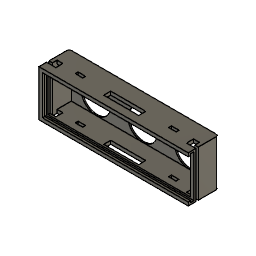
Canal - base v22 (Autodesk Fusion 360 design; units mm, degrees)
Autodesk Fusion 360 part; units mm, degrees
sketch "Esquisse1" plane through (0, 0, 0) normal (0, 1, 0) x (1, 0, 0)
  line L0 (-18.0113, -0.0987) -> (45.9887, -0.0987)
  line L1 (45.9887, -0.0987) -> (45.9887, -19.8487)
  line L2 (45.9887, -19.8487) -> (-18.0113, -19.8487)
  line L3 (-18.0113, -19.8487) -> (-18.0113, -0.0987)
  dimension "d1" = 64
  dimension "d2" = 19.75
  constraint horizontal L0
  constraint vertical L1
  constraint horizontal L2
  constraint vertical L3
  measures "d1" distance of L1 L3
  measures "d2" distance of L0 L2
extrude "Extrusion1" add sketch "Esquisse1" along normal blind 13
shell "Coque2" thickness 1.5 removed faces 1 at (3.3221, 0, 6.682)
sketch "Esquisse3" plane through (0, 0, 0.0987) normal (0, 0, -1) x (1, 0, 0)
  line L0 (45.9887, 0) -> (-18.0113, 0)
  line L1 (-18.0113, 0) -> (-18.0113, -13)
  line L2 (-18.0113, -13) -> (45.9887, -13)
  line L3 (45.9887, -13) -> (45.9887, 0)
  line L4 (21.4887, -6.3) -> (6.4887, -6.3)
  line L5 (6.4887, -6.3) -> (6.4887, -3.3)
  line L6 (6.4887, -3.3) -> (21.4887, -3.3)
  line L7 (21.4887, -3.3) -> (21.4887, -6.3)
  line L8 (13.9887, -13) -> (13.9887, 0) construction
  dimension "d12" = 3
  dimension "d14" = 15
  dimension "d57" = 6.7
  constraint horizontal L4
  constraint vertical L5
  constraint horizontal L6
  constraint vertical L7
  constraint midpoint L2 L8.start
  constraint midpoint L0 L8.end
  constraint symmetric L5 L7 L8
  measures "d12" distance of L4 L6
  measures "d14" distance of L5 L7
  measures "d57" distance of L2 L4
extrude "Extrusion3" cut sketch "Esquisse3" against normal blind 25 contours L4 L5 L6 L7
sketch "Esquisse4" plane through (0, 0, 0) normal (0, 0, 1) x (1, 0, 0)
sketch "Esquisse8" plane through (0, 11.5, 0) normal (0, -1, 0) x (1, 0, 0)
  line L0 (44.4887, 18.3487) -> (-16.5113, 18.3487)
  line L1 (-16.5113, 18.3487) -> (-16.5113, 1.5987)
  line L2 (-16.5113, 1.5987) -> (44.4887, 1.5987)
  line L3 (44.4887, 1.5987) -> (44.4887, 18.3487)
  line L4 (-16.5113, 18.3487) -> (44.4887, 18.3487)
  line L5 (44.4887, 18.3487) -> (44.4887, 1.5987)
  line L6 (44.4887, 1.5987) -> (-16.5113, 1.5987)
  line L7 (-16.5113, 1.5987) -> (-16.5113, 18.3487)
  constraint horizontal L4
  constraint vertical L5
  constraint horizontal L6
  constraint vertical L7
  constraint coincident L2.end L3.start
  constraint coincident L0.end L1.start
extrude "Extrusion5" cut sketch "Esquisse8" against normal blind 0.9
sketch "Esquisse9" plane through (0, 13, 0) normal (0, 1, 0) x (-1, 0, 0)
  line L0 (18.0113, 19.8487) -> (-45.9887, 19.8487)
  line L1 (-45.9887, 19.8487) -> (-45.9887, 0.0987)
  line L2 (-45.9887, 0.0987) -> (18.0113, 0.0987)
  line L3 (18.0113, 0.0987) -> (18.0113, 19.8487)
  circle A0 centre (6.0113, 7.8487) radius 6.25
  circle A1 centre (-13.9887, 7.8487) radius 6.25
  circle A2 centre (-33.9887, 7.8487) radius 6.25
  dimension "d25" = 12.5
  dimension "d26" = 12
  dimension "d29" = -40
  dimension "d30" = 0
  dimension "d56" = 7.75
  measures "d25" diameter of A0
  measures "d26" distance of L3 A0.centre
  measures "d56" distance of L2 A0.centre
extrude "Extrusion6" cut sketch "Esquisse9" against normal blind 1 contours A0 | A1 | A2
ref_plane "Plan de construction1" through (13.9887, 6.2, 9.9737) normal (0, 0, 1) x (1, 0, 0)
sketch "Esquisse10" plane through (0, 0, 18.3487) normal (0, 0, -1) x (1, 0, 0)
  line L0 (6.4887, -6.3) -> (6.4887, -3.3)
  line L1 (6.4887, -3.3) -> (21.4887, -3.3)
  line L2 (21.4887, -3.3) -> (21.4887, -6.3)
  line L3 (21.4887, -6.3) -> (6.4887, -6.3)
  line L4 (44.4887, 0) -> (-16.5113, 0)
  line L5 (-16.5113, 0) -> (-16.5113, -12.4)
  line L6 (-16.5113, -12.4) -> (44.4887, -12.4)
  line L7 (44.4887, -12.4) -> (44.4887, 0)
  line L8 (-7.6113, -5.2) -> (-4.4113, -5.2)
  line L9 (-4.4113, -5.2) -> (-4.4113, -6.4)
  line L10 (-4.4113, -6.4) -> (-7.6113, -6.4)
  line L11 (-7.6113, -6.4) -> (-7.6113, -5.2)
  line L12 (13.9887, 0) -> (13.9887, -10.4) construction
  line L13 (-6.0113, -5.2) -> (-6.0113, -6.4) construction
  line L14 (35.5887, -6.4) -> (35.5887, -5.2)
  line L15 (35.5887, -5.2) -> (32.3887, -5.2)
  line L16 (32.3887, -5.2) -> (32.3887, -6.4)
  line L17 (32.3887, -6.4) -> (35.5887, -6.4)
  line L18 (45.9887, -13) -> (-18.0113, -13)
  dimension "d33" = 3.2
  dimension "d34" = 1.2
  dimension "d36" = 20
  dimension "d58" = 6.6
  constraint horizontal L8
  constraint vertical L9
  constraint horizontal L10
  constraint vertical L11
  constraint midpoint L4 L12.start
  constraint perpendicular L6 L12
  constraint midpoint L8 L13.start
  constraint midpoint L10 L13.end
  constraint symmetric L8.start L12 L14.end
  constraint symmetric L8.end L12 L15.end
  constraint symmetric L9.end L12 L16.end
  constraint symmetric L10.end L12 L14.start
  measures "d33" distance of L9 L11
  measures "d34" distance of L8 L10
  measures "d36" distance of L12 L13
  measures "d58" distance of L10 L18
extrude "Extrusion7" cut sketch "Esquisse10" against normal blind 2 contours L8 L9 L10 L11 | L14 L15 L16 L17
mirror "Symétrie miroir1" about plane through (13.9887, 6.2, 9.9737) normal (0, 0, 1) of "Extrusion7"
sketch "Esquisse11" plane through (45.9887, 0, 0) normal (1, 0, 0) x (0, 1, 0)
  line L0 (0, 19.8487) -> (0, 0.0987)
  line L1 (0, 0.0987) -> (13, 0.0987)
  line L2 (13, 0.0987) -> (13, 19.8487)
  line L3 (13, 19.8487) -> (0, 19.8487)
  line L4 (1, 19.0487) -> (2.4, 19.0487)
  line L5 (2.4, 19.0487) -> (2.4, 0.8987)
  line L6 (2.4, 0.8987) -> (1, 0.8987)
  line L7 (1, 0.8987) -> (1, 19.0487)
  line L8 (0, 9.9737) -> (13, 9.9737) construction
  dimension "d41" = 1.4
  dimension "d42" = 1
  dimension "d43" = 0.8
  constraint horizontal L4
  constraint vertical L5
  constraint horizontal L6
  constraint vertical L7
  constraint midpoint L0 L8.start
  constraint midpoint L2 L8.end
  constraint symmetric L4 L6 L8
  measures "d41" distance of L5 L7
  measures "d42" distance of L0 L7
  measures "d43" distance of L1 L6
extrude "Extrusion8" cut sketch "Esquisse11" against normal blind 63.2 contours L4 L5 L6 L7
sketch "Esquisse12" plane through (0, 0, 0) normal (0, -1, 0) x (1, 0, 0)
  line L0 (-16.5113, 1.5987) -> (-16.5113, 18.3487)
  line L1 (-16.5113, 18.3487) -> (44.4887, 18.3487)
  line L2 (44.4887, 18.3487) -> (44.4887, 1.5987)
  line L3 (44.4887, 1.5987) -> (-16.5113, 1.5987)
  line L4 (45.9887, 19.8487) -> (-18.0113, 19.8487)
  line L5 (-18.0113, 19.8487) -> (-18.0113, 0.0987)
  line L6 (-18.0113, 0.0987) -> (45.9887, 0.0987)
  line L7 (45.9887, 0.0987) -> (45.9887, 19.8487)
  line L8 (44.4887, 1.5987) -> (45.9887, 1.5987)
  line L9 (44.4887, 18.3487) -> (45.9887, 18.3487)
  constraint coincident L2.end L3.start
  constraint coincident L7 L8.end
  constraint perpendicular L7 L8
  constraint coincident L1.end L2.start
  constraint coincident L7 L9.end
  constraint perpendicular L7 L9
extrude "Extrusion9" cut sketch "Esquisse12" against normal blind 1 contours L2 L7 L8 L9
sketch "Esquisse15" plane through (0, 0, 0.0987) normal (0, 0, -1) x (1, 0, 0)
  line L0 (-4.4113, -5.2) -> (-4.4113, -6.4)
  line L1 (-4.4113, -6.4) -> (-7.6113, -6.4)
  line L2 (-7.6113, -6.4) -> (-7.6113, -5.2)
  line L3 (-7.6113, -5.2) -> (-4.4113, -5.2)
  line L4 (35.5887, -5.2) -> (35.5887, -6.4)
  line L5 (35.5887, -6.4) -> (32.3887, -6.4)
  line L6 (32.3887, -6.4) -> (32.3887, -5.2)
  line L7 (32.3887, -5.2) -> (35.5887, -5.2)
  line L8 (6.4887, -6.3) -> (6.4887, -3.3)
  line L9 (6.4887, -3.3) -> (21.4887, -3.3)
  line L10 (21.4887, -3.3) -> (21.4887, -6.3)
  line L11 (21.4887, -6.3) -> (6.4887, -6.3)
  line L12 (45.9887, 0) -> (-18.0113, 0)
  line L13 (-18.0113, 0) -> (-18.0113, -13)
  line L14 (-18.0113, -13) -> (45.9887, -13)
  line L15 (45.9887, -13) -> (45.9887, 0)
  line L16 (45.9887, -3.3) -> (41.9887, -3.3)
  line L17 (41.9887, -3.3) -> (41.9887, -6.3)
  line L18 (41.9887, -6.3) -> (44.4887, -6.3)
  line L19 (44.4887, -6.3) -> (44.4887, -4.3)
  line L20 (44.4887, -4.3) -> (45.9887, -4.3)
  line L21 (13.9887, 0) -> (13.9887, -13) construction
  line L22 (-16.5113, -4.3) -> (-18.0113, -4.3)
  line L23 (-16.5113, -6.3) -> (-16.5113, -4.3)
  line L24 (-14.0113, -6.3) -> (-16.5113, -6.3)
  line L25 (-14.0113, -3.3) -> (-14.0113, -6.3)
  line L26 (-18.0113, -3.3) -> (-14.0113, -3.3)
  dimension "d49" = 1
  dimension "d50" = 1.5
  dimension "d51" = 2.5
  dimension "d52" = 3
  dimension "d59" = 0.1
  constraint coincident L15 L16.start
  constraint perpendicular L15 L16
  constraint perpendicular L16 L17
  constraint perpendicular L17 L18
  constraint perpendicular L18 L19
  constraint coincident L15 L20.end
  constraint perpendicular L15 L20
  constraint midpoint L12 L21.start
  constraint midpoint L14 L21.end
  constraint symmetric L16.start L21 L26.start
  constraint symmetric L16.end L21 L25.start
  constraint symmetric L17.end L21 L24.start
  constraint symmetric L18.end L21 L23.start
  constraint symmetric L19.end L21 L22.start
  constraint symmetric L20.end L21 L22.end
  measures "d49" distance of L16 L20
  measures "d50" distance of L15 L19
  measures "d51" distance of L17 L19
  measures "d52" distance of L16 L18
  measures "d59" distance of L5 L18
extrude "Extrusion10" cut sketch "Esquisse15" against normal blind 31 contours L15 L16 L17 L18 L19 L20 | L13 L22 L23 L24 L25 L26
fillet "Fillet1" radius 1 2 edges at (45.9887, 13, 9.9737) (-18.0113, 13, 9.9737)
